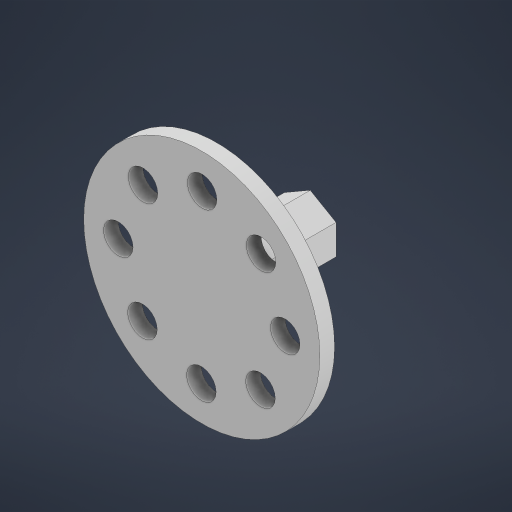
# Autodesk Inventor part: ArmInsert
Saved by Autodesk Inventor 2023 (Build 270158000, 158)
## iProperties
Created: 2023-12-24
Part Number: ArmInsert
Material: Generic
Document SubType Name: Modeling
Designer: kelle
Density: 1 g/cm^3
Appearance: Default
Author: kelle
Autodesk Inventor part; units mm, degrees
ref_plane "YZ Plane" through (0, 0, 0) normal (1, 0, 0) x (0, 1, 0)
ref_plane "XZ Plane" through (0, 0, 0) normal (0, 1, 0) x (-1, 0, 0)
ref_plane "XY Plane" through (0, 0, 0) normal (0, 0, 1) x (1, 0, 0)
sketch "Sketch1" plane through (0, 0, 0) normal (0, 0, 1) x (1, 0, 0)
  line L0 (-3.5, 2.0207) -> (0, 4.0415)
  line L1 (0, 4.0415) -> (3.5, 2.0207)
  line L2 (3.5, 2.0207) -> (3.5, -2.0207)
  line L3 (3.5, -2.0207) -> (0, -4.0415)
  line L4 (0, -4.0415) -> (-3.5, -2.0207)
  line L5 (-3.5, -2.0207) -> (-3.5, 2.0207)
  point P0 (0, 0)
  point P1 (0, 0)
  dimension "d0" = 7
  constraints: 12 end point, 1 coincident, 13 other
  measures "d0" distance between parallel lines of L2 L5
extrude "Extrusion1" add sketch "Sketch1" along normal blind 12.7
sketch "Sketch2" plane through (0, 0, 12.7) normal (0, 0, 1) x (1, 0, 0)
  line L0 (-11.3137, 0.0513) -> (-7.9637, 8.0363) construction
  line L1 (-7.9637, 8.0363) -> (0.0513, 11.3137) construction
  line L2 (0.0513, 11.3137) -> (8.0363, 7.9637) construction
  line L3 (8.0363, 7.9637) -> (11.3137, -0.0513) construction
  line L4 (11.3137, -0.0513) -> (7.9637, -8.0363) construction
  line L5 (7.9637, -8.0363) -> (-0.0513, -11.3137) construction
  line L6 (-0.0513, -11.3137) -> (-8.0363, -7.9637) construction
  line L7 (-8.0363, -7.9637) -> (-11.3137, 0.0513) construction
  circle A0 centre (0, 0) radius 16
  circle A1 centre (-7.9637, 8.0363) radius 2
  circle A2 centre (-11.3137, 0.0513) radius 2
  circle A3 centre (-8.0363, -7.9637) radius 2
  circle A4 centre (-0.0513, -11.3137) radius 2
  circle A5 centre (7.9637, -8.0363) radius 2
  circle A6 centre (11.3137, -0.0513) radius 2
  circle A7 centre (8.0363, 7.9637) radius 2
  circle A8 centre (0.0513, 11.3137) radius 2
  dimension "d3" = 16
  dimension "d4" = 32
  dimension "d5" = 4
  dimension "d8" = 360
  constraints: 16 end point, 9 centre point, 3 coincident, 34 other
  measures "d3" horizontal distance of L2.end L0.end
  measures "d4" diameter of A0
  measures "d5" diameter of A1
extrude "Extrusion2" add sketch "Sketch2" along normal blind 2
body "Solid1"
